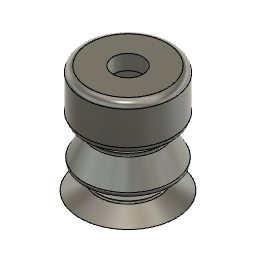
StyloVentouse v8 (Autodesk Fusion 360 archive; units mm, degrees)
design "VENTOUSE_15MM"
Autodesk Fusion 360 part; units mm, degrees
note: some values were not read from the file. Chosen so that the rebuilt part matches the saved one: which face or edge a step refers to; where a thread starts. Set by a fixed rule: which sketch regions a step uses.
sketch "Sketch1" plane through (0, 0, 0) normal (0, 1, 0) x (1, 0, 0)
sketch "Sketch2" plane through (0, 0, 0) normal (1, 0, 0) x (0, 0, -1)
  line L0 (8, 0) -> (4.6728, 1.6982)
  line L1 (4.6728, 1.6982) -> (7.5, 4.5279)
  line L2 (7.5, 4.5279) -> (5.2639, 9)
  line L3 (5.2639, 9) -> (7.5, 11)
  line L4 (7.5, 11) -> (7.5, 18)
  line L5 (7.5, 18) -> (2.5, 18)
  line L6 (2.5, 18) -> (2.5, 15.5)
  line L7 (2.5, 15.5) -> (4, 15.5)
  line L8 (4, 15.5) -> (4, 13.2)
  line L9 (4, 13.2) -> (2.5, 13.2)
  line L10 (2.5, 13.2) -> (2.5, 9)
  line L11 (2.5, 9) -> (6.2834, 4.725)
  line L12 (6.2834, 4.725) -> (4, 1.6283)
  line L13 (4, 1.6283) -> (8, 0)
  line L14 (0, 0) -> (0, 19.3777) construction
  dimension "d1" = 7.5
  dimension "d2" = 2.5
  dimension "d3" = 8
  dimension "d5" = 18
  dimension "d6" = 2.3
  dimension "d8" = 3
  dimension "d9" = 5
  dimension "d10" = 4
  dimension "d11" = 7
  dimension "d14" = 2.5
  dimension "d15" = 4
  dimension "d19" = 2
  dimension "d20" = 1
  dimension "d21" = 4
  dimension "d22" = 0.5
  dimension "d23" = 0.3681
  dimension "d24" = 1
  constraint vertical L4
  constraint perpendicular L4 L5
  constraint perpendicular L5 L6
  constraint perpendicular L6 L7
  constraint perpendicular L7 L8
  constraint perpendicular L8 L9
  constraint perpendicular L9 L10
  constraint collinear L6 L10
  constraint horizontal L0.start L14.start
  constraint horizontal L2.end L10.end
  constraint vertical L1.end L3.end
  constraint coincident L14.start origin
  constraint vertical L14
  measures "d1" distance of L14.start L4
  measures "d2" distance of L14.start L6
  measures "d3" distance of L0.start L14.start
  measures "d5" distance of L14.start L5
  measures "d6" distance of L7.end L8.end
  measures "d8" distance of L2.end L3.end
  measures "d9" distance of L1.end L2.end
  measures "d10" distance of L0.end L1.end
  measures "d11" distance of L3.end L4.end
  measures "d14" distance of L5.end L6.end
  measures "d15" distance of L8 L14.start
  measures "d19" vertical distance of L2.end L3.end
  measures "d20" distance of L2 L11.end
  measures "d21" horizontal distance of L12.end L14.start
  measures "d22" distance of L0.end L12
  measures "d23" distance of L0 L12.end
  measures "d24" distance of L1 L11.end
revolve "Revolve1" add sketch "Sketch2" angle 360 about axis through (0, 0, 0) along (0, 1, 0)
fillet "Fillet1" radius 1 1 edges at (-6.9925, 18, -2.7121)
fillet "Fillet2" radius 1 1 edges at (-6.9925, 11, -2.7121)
fillet "Fillet2" radius 0.5 1 edges at (-6.9925, 4.5279, -2.7121)
fillet "Fillet3" radius 0.25 1 edges at (-4.3565, 1.6982, -1.6897)
fillet "Fillet4" radius 0.5 1 edges at (-4.9077, 9, -1.9035)

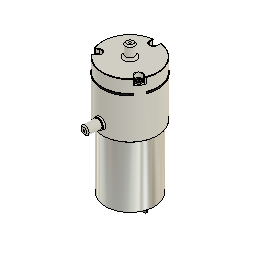
design "MICRO-POMPE 370"
Autodesk Fusion 360 part; units mm, degrees
sketch "Sketch1" plane through (0, 0, 0) normal (0, 0, 1) x (1, 0, 0)
  circle A0 centre (0, 0) radius 12.05
  dimension "d1" = 24.1
  measures "d1" diameter of A0
extrude "Extrude1" add sketch "Sketch1" along normal blind 30.9 makes body 1 in component "MOTEUR"
sketch "Sketch1 (2)" plane through (0, 0, 0) normal (0, 0, -1) x (1, 0, 0) in component "MOTEUR"
  circle A0 centre (0, 0) radius 12.05
  circle A1 centre (0, 0) radius 11.55
  dimension "d4" = 0.5
  measures "d4" distance of A0 A1
extrude "Extrude2" cut sketch "Sketch1 (2)" against normal blind 0.8 contours A1 bodies 1 in component "MOTEUR"
sketch "Sketch2" plane through (0, 0, 0.8) normal (0, 0, -1) x (1, 0, 0) in component "MOTEUR"
  circle A0 centre (0, 0) radius 11.55
  circle A1 centre (0, 0) radius 3.3
  dimension "d7" = 6.6
  measures "d7" diameter of A1
extrude "Extrude3" add sketch "Sketch2" along normal blind 2.3 contours A1 bodies 1 in component "MOTEUR"
fillet "Fillet1" radius 1 1 edges at (-3.0767, 1.1933, -1.5) on bodies 1 in component "MOTEUR"
sketch "Sketch3" plane through (0, 0, 0.8) normal (0, 0, -1) x (1, 0, 0) in component "MOTEUR"
  circle A0 centre (0, 0) radius 3.3
  circle A1 centre (0, 0) radius 11.55
  line L0 (0, 0) -> (9, 0) construction
  line L1 (10.8, -2) -> (10.8, 2)
  arc A2 (10.8, 2) -> (7.2, 2) centre (9, 2) ccw
  line L2 (7.2, 2) -> (7.2, -2)
  arc A3 (7.2, -2) -> (10.8, -2) centre (9, -2) ccw
  line L3 (9, -2) -> (9, 2) construction
  dimension "d11" = 9
  dimension "d12" = 4
  dimension "d13" = 1.8
  measures "d11" distance of A0.centre
  measures "d13" radius of A2
extrude "Extrude1'" add sketch "Sketch3" along normal blind 0.5 separate body contours L1 A2 L2 A3 makes body 2 in component "PAD_MOTEUR"
mirror "MirrorComponent1" about plane through (0, 0, 0) normal (0, 0, 1) of bodies 2 makes body 3 in component "PAD_MOTEUR(Mirror)"
sketch "Sketch4" plane through (0, 0, 0.8) normal (0, 0, -1) x (1, 0, 0) in component "MOTEUR"
  circle A0 centre (0, 0) radius 3.3
  circle A1 centre (0, 0) radius 11.55
  line L0 (-8, -2) -> (-10, -2)
  line L1 (-10, -2) -> (-10, -1.5)
  line L2 (-10, -1.5) -> (-8, -1.5)
  line L3 (-8, -1.5) -> (-8, -2)
  line L4 (-8, -2) -> (-10, -1.5) construction
  line L5 (-10, -2) -> (-8, -1.5) construction
  arc A2 (-7.2, 2) -> (-10.8, 2) centre (-9, 2) ccw
  line L6 (-9, -1.75) -> (-9, 3.8)
  dimension "d16" = 0.5
  dimension "d17" = 2
extrude "Extrude1''" add sketch "Sketch4" along normal blind 4 separate body contours L0 L1 L2 L3 makes body 4 in component "PIN"
fillet "Fillet1'" radius 0.5 2 edges at (-8, 1.75, -3.2) (-10, 1.75, -3.2) on bodies 4 in component "PIN"
other "C-Pattern1" in component "MOTEUR"
sketch "Sketch2 (2)" plane through (0, 0, 30.9) normal (0, 0, 1) x (-1, 0, 0)
  circle A0 centre (0, 0) radius 12.05
  circle A1 centre (0, 0) radius 13.55
  dimension "d23" = 27.1
  measures "d23" diameter of A1
extrude "Extrude1'''" add sketch "Sketch2 (2)" along normal blind 27.1 separate body contours A0 | A1 makes body 5 in component "CORPS"
sketch "Sketch1 (3)" plane through (0, 0, 58) normal (0, 0, 1) x (-1, 0, 0) in component "CORPS"
  circle A0 centre (0, 0) radius 13.55
  line L0 (0, 0) -> (0, -13.55) construction
  line L1 (1.75, -13.55) -> (1.75, -11.55)
  arc A1 (1.75, -11.55) -> (-1.75, -11.55) centre (0, -11.55) ccw
  line L2 (-1.75, -11.55) -> (-1.75, -13.55)
  arc A2 (-1.75, -13.55) -> (1.75, -13.55) centre (0, -13.55) ccw
  line L3 (0, -13.55) -> (0, -11.55) construction
  dimension "d26" = 2
  dimension "d27" = 3.5
  measures "d27" distance of L1 L2
extrude "Extrude2'" cut sketch "Sketch1 (3)" against normal blind 3 contours A0 L1 A1 L2 picked at (0.1949, -12.2125) bodies 5 in component "CORPS"
pattern_circular "C-Pattern1'" count 3 over 360 about axis through (0, 0, 30.9) along (0, 0, 1) of "Extrude2'" in component "CORPS"
sketch "Sketch2 (3)" plane through (0, 0, 58) normal (0, 0, 1) x (-1, 0, 0) in component "CORPS"
  line L0 (-10.7614, 8.2338) -> (-9.1276, 7.2905)
  arc A0 (-10.8776, 4.2595) -> (-9.1276, 7.2905) centre (-10.0026, 5.775) ccw
  line L1 (-10.8776, 4.2595) -> (-12.5114, 5.2027)
  arc A1 (-12.5114, 5.2027) -> (-1.75, -13.4365) centre (0, 0) ccw
  line L2 (-1.75, -13.4365) -> (-1.75, -11.55)
  arc A2 (1.75, -11.55) -> (-1.75, -11.55) centre (0, -11.55) ccw
  line L3 (1.75, -11.55) -> (1.75, -13.4365)
  arc A3 (1.75, -13.4365) -> (12.5114, 5.2027) centre (0, 0) ccw
  line L4 (12.5114, 5.2027) -> (10.8776, 4.2595)
  arc A4 (9.1276, 7.2905) -> (10.8776, 4.2595) centre (10.0026, 5.775) ccw
  line L5 (9.1276, 7.2905) -> (10.7614, 8.2338)
  arc A5 (10.7614, 8.2338) -> (-10.7614, 8.2338) centre (0, 0) ccw
  circle A6 centre (0, 0) radius 2.15
  dimension "d32" = 4.3
  measures "d32" diameter of A6
extrude "Extrude3'" add sketch "Sketch2 (3)" along normal blind 6.1 contours A6 bodies 5 in component "CORPS"
sketch "Sketch3 (2)" plane through (0, 0, 64.1) normal (0, 0, 1) x (-1, 0, 0) in component "CORPS"
  circle A0 centre (0, 0) radius 2.15
  circle A1 centre (0, 0) radius 0.5
  dimension "d35" = 1
  measures "d35" diameter of A1
extrude "Extrude4" cut sketch "Sketch3 (2)" against normal blind 6 contours A1 bodies 5 in component "CORPS"
fillet "Fillet1''" radius 1 1 edges at (2.0045, -0.7775, 58) on bodies 5 in component "CORPS"
fillet "Fillet2" radius 0.4 6 edges at (10.7614, -8.2338, 56.5) (12.5114, -5.2027, 56.5) (-10.7614, -8.2338, 56.5) (-12.5114, -5.2027, 56.5) (-1.75, 13.4365, 56.5) (1.75, 13.4365, 56.5) on bodies 5 in component "CORPS"
sketch "Sketch4 (2)" plane through (0, 0, 55) normal (0, 0, 1) x (-1, 0, 0) in component "CORPS"
  arc A0 (-2.2154, -13.3677) -> (2.2154, -13.3677) centre (0, 0) ccw
  arc A1 (1.75, -12.973) -> (2.2154, -13.3677) centre (2.15, -12.973) ccw
  line L0 (1.75, -12.973) -> (1.75, -11.55)
  arc A2 (1.75, -11.55) -> (-1.75, -11.55) centre (0, -11.55) ccw
  line L1 (-1.75, -11.55) -> (-1.75, -12.973)
  arc A3 (-2.2154, -13.3677) -> (-1.75, -12.973) centre (-2.15, -12.973) ccw
  circle A4 centre (0, -11.55) radius 1.5
  dimension "d41" = 3
  measures "d41" diameter of A4
extrude "Extrude1''''" add sketch "Sketch4 (2)" along normal blind 1.2 separate body contours A4 makes body 6 in component "VIS"
sketch "Sketch1 (4)" plane through (0, 0, 56.2) normal (0, 0, 1) x (-1, 0, 0) in component "VIS"
  circle A0 centre (0, -11.55) radius 1.5
  line L0 (-0.2169, -12.6709) -> (0.2169, -12.6709)
  line L1 (0.2169, -12.6709) -> (0.2169, -10.4291)
  line L2 (0.2169, -10.4291) -> (-0.2169, -10.4291)
  line L3 (-0.2169, -10.4291) -> (-0.2169, -12.6709)
  line L4 (-0.2169, -12.6709) -> (0.2169, -10.4291) construction
  line L5 (0.2169, -12.6709) -> (-0.2169, -10.4291) construction
  line L6 (-1.113, -11.7669) -> (1.113, -11.7669)
  line L7 (1.113, -11.7669) -> (1.113, -11.3331)
  line L8 (1.113, -11.3331) -> (-1.113, -11.3331)
  line L9 (-1.113, -11.3331) -> (-1.113, -11.7669)
  line L10 (-1.113, -11.7669) -> (1.113, -11.3331) construction
  line L11 (1.113, -11.7669) -> (-1.113, -11.3331) construction
extrude "Extrude2''" cut sketch "Sketch1 (4)" against normal blind 0.35 contours L0 L1 L3 L6 | L3 L6 L8 L9 | L1 L3 L6 L8 | L1 L6 L7 L8 | L1 L2 L3 L8 bodies 6 in component "VIS"
fillet "Fillet1'''" radius 0.2 2 edges at (1.3985, 12.0924, 55) (1.3985, 12.0924, 56.2) on bodies 6 in component "VIS"
other "C-Pattern1''" in component "CORPS"
ref_plane "WorkPlane1" through (0, 0, 12.125) normal (0.087156, 0.996195, 0) x (0, 0, 1) in component "CORPS"
sketch "Sketch5" plane through (0, 0, 12.125) normal (0.087156, 0.996195, 0) x (0, 0, 1) in component "CORPS"
  line L0 (18.775, -13.55) -> (18.775, 13.55)
  line L1 (18.775, 0) -> (23.775, 0) construction
  circle A0 centre (23.775, 0) radius 2.6631
  dimension "d50" = 5
  dimension "d51" = 5.3262
  measures "d50" distance of origin
  measures "d51" diameter of A0
extrude "Extrude5" add sketch "Sketch5" against normal blind 14.5 bodies 5 in component "CORPS"
sketch "Sketch6" plane through (-1.2638, -14.4448, 0) normal (-0.087156, -0.996195, 0) x (0.996195, -0.087156, 0) in component "CORPS"
  circle A0 centre (0, 35.9) radius 2.6631
  circle A1 centre (0, 35.9) radius 2.1
  circle A2 centre (0, 35.9) radius 0.5
  dimension "d54" = 4.2
  dimension "d55" = 1
  measures "d54" diameter of A1
  measures "d55" diameter of A2
extrude "Extrude6" add sketch "Sketch6" along normal blind 6.5 contours A1 bodies 5 in component "CORPS"
chamfer "Chamfer1" distance 0.6 angle 45 2 edges at (2.0045, 0.7775, 64.1) (-3.7807, -20.7494, 35.1406) on bodies 5 in component "CORPS"
fillet "Fillet3" radius 0.1 1 edges at (-0.3044, -14.5288, 33.4171) on bodies 5 in component "CORPS"
fillet "Fillet4" radius 0.2 19 edges at (10.5536, -8.277, 58) (9.7438, -7.6463, 58) (8.487, -4.9, 58) (11.4938, -4.6152, 58) (12.4449, -5.0011, 58) (11.7346, 6.775, 58) (1.8913, 13.2781, 58) (1.75, 12.2615, 58) (0, 9.8, 58) (-1.75, 12.2615, 58) (-1.8913, 13.2781, 58) (-11.7346, 6.775, 58) (-12.4449, -5.0011, 58) (-11.4938, -4.6152, 58) (-8.487, -4.9, 58) (-9.7438, -7.6463, 58) (-10.5536, -8.277, 58) (0, -13.55, 58) (12.633, 4.8999, 30.9) on bodies 5 in component "CORPS"
ref_plane "WorkPlane2" through (0, -0.0822, 50.8) normal (0, 0, 1) x (-1, 0, 0) in component "CORPS"
sketch "Sketch8" plane through (0, -0.0822, 50.8) normal (0, 0, 1) x (1, 0, 0) in component "CORPS"
  circle A0 centre (0, 0.0822) radius 13.65
  line L0 (0, 0.0822) -> (-12.7781, -4.7182)
  line L1 (0, 0.0822) -> (-2.2317, 13.5486)
  dimension "d61" = 27.3
  measures "d61" diameter of A0
extrude "Extrude1'''''" add sketch "Sketch8" along normal blind 1 separate body contours A0 L0 L1 picked at (-8.7073, -2.4762) makes body 7 in component "JOINT"
fillet "Fillet1''''" radius 0.1 2 edges at (-11.8212, 6.825, 51.8) (-11.8212, 6.825, 50.8) on bodies 7 in component "JOINT"
other "C-Pattern2" in component "CORPS"
component "MOTEUR" placed x (1, 0, 0) y (0, 1, 0) z (0, 0, 1) at (0, 0, 0)
component "CORPS" placed x (1, 0, 0) y (0, 1, 0) z (0, 0, 1) at (0, 0, 0)
component "PAD_MOTEUR" placed x (1, 0, 0) y (0, 1, 0) z (0, 0, 1) at (0, 0, 0) in component "MOTEUR"
component "PAD_MOTEUR(Mirror)" placed x (-1, 0, 0) y (0, 1, 0) z (0, 0, -1) at (0, 0, 0) in component "MOTEUR"
component "PIN" placed x (1, 0, 0) y (0, 1, 0) z (0, 0, 1) at (0, 0, 0) in component "MOTEUR"
component "PIN" placed x (-1, 0, 0) y (0, -1, 0) z (0, 0, 1) at (0, 0, 0) in component "MOTEUR"
component "VIS" placed x (1, 0, 0) y (0, 1, 0) z (0, 0, 1) at (0, 0, 0) in component "CORPS"
component "VIS" placed x (-0.5, 0.866025, 0) y (-0.866025, -0.5, 0) z (0, 0, 1) at (0, 0, 0) in component "CORPS"
component "VIS" placed x (-0.5, -0.866025, 0) y (0.866025, -0.5, 0) z (0, 0, 1) at (0, 0, 0) in component "CORPS"
component "JOINT" placed x (1, 0, 0) y (0, 1, 0) z (0, 0, 1) at (0, 0, 0) in component "CORPS"
component "JOINT" placed x (-0.5, 0.866025, 0) y (-0.866025, -0.5, 0) z (0, 0, 1) at (0, 0, 0) in component "CORPS"
component "JOINT" placed x (-0.5, -0.866025, 0) y (0.866025, -0.5, 0) z (0, 0, 1) at (0, 0, 0) in component "CORPS"
equation "d52 = -( ( 27 / 2 ) * 1 mm ) - 1 mm"

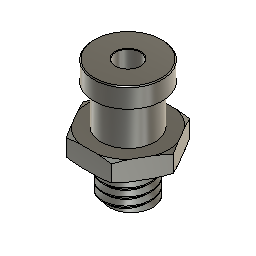
design "RACCORD-VENTOUSE"
Autodesk Fusion 360 part; units mm, degrees
sketch "Sketch1" plane through (0, 0, 0) normal (1, 0, 0) x (0, 1, 0)
  line L0 (0, 0) -> (3.5, 0)
  line L1 (3.5, 0) -> (3.5, -2)
  line L2 (3.5, -2) -> (2.75, -2)
  line L3 (2.75, -2) -> (2.75, -6)
  line L4 (2.75, -6) -> (0, -6)
  line L5 (0, -6) -> (0, 0)
  dimension "d1" = 3.5
  dimension "d2" = 2.75
  dimension "d3" = 2
  dimension "d4" = 4
  measures "d1" distance of L0.start
  measures "d2" distance of L3 L5
revolve "Revolve1" add sketch "Sketch1" angle 360 about axis through (0, 0, -6) along (0, 0, 1)
sketch "Sketch2" plane through (0, 0, -6) normal (0, 0, -1) x (1, 0, 0)
  circle A0 centre (0, 0) radius 2.75
  line L0 (2.3094, -4) -> (4.6188, 0)
  line L1 (4.6188, 0) -> (2.3094, 4)
  line L2 (2.3094, 4) -> (-2.3094, 4)
  line L3 (-2.3094, 4) -> (-4.6188, 0)
  line L4 (-4.6188, 0) -> (-2.3094, -4)
  line L5 (-2.3094, -4) -> (2.3094, -4)
  dimension "d6" = 8
  measures "d6" distance of L2 L5
extrude "Extrude1" add sketch "Sketch2" along normal blind 2 contours A0 | L0 L1 L2 L3 L4 L5
sketch "Sketch3" plane through (0, 0, 0) normal (0, 1, 0) x (1, 0, 0)
  line L0 (4.6188, 6) -> (2.3094, 6) construction
  line L1 (4.6188, 6) -> (4.6188, 8) construction
  line L2 (4.1193, 6) -> (4.6188, 6.1563)
  line L3 (4.6188, 6) -> (4.1193, 6)
  line L4 (4.6188, 8) -> (2.3094, 8) construction
  line L5 (4.6188, 7.8437) -> (4.1193, 8)
  line L6 (4.1193, 8) -> (4.6188, 8)
  line L7 (4.6188, 7.8437) -> (4.6188, 8)
  line L8 (4.6188, 6) -> (4.6188, 6.1563)
revolve "Revolve2" cut sketch "Sketch3" angle 360 about axis through (0, 0, 1.75) along (0, 0, 1)
chamfer "Chamfer1" distance 0.1 angle 45 1 edges at (-3.2631, 1.2657, 0)
sketch "Sketch4" plane through (0, 0, -8) normal (0, 0, -1) x (1, 0, 0)
  arc A0 (-3.9563, 1.1475) -> (-3.9563, -1.1475) centre (0, 0) ccw
  line L0 (-3.9563, -1.1475) -> (-2.9719, -2.8525)
  arc A1 (-2.9719, -2.8525) -> (-0.9843, -4) centre (0, 0) ccw
  line L1 (-0.9843, -4) -> (0.9843, -4)
  arc A2 (0.9843, -4) -> (2.9719, -2.8525) centre (0, 0) ccw
  line L2 (2.9719, -2.8525) -> (3.9563, -1.1475)
  arc A3 (3.9563, -1.1475) -> (3.9563, 1.1475) centre (0, 0) ccw
  line L3 (3.9563, 1.1475) -> (2.9719, 2.8525)
  arc A4 (2.9719, 2.8525) -> (0.9843, 4) centre (0, 0) ccw
  line L4 (0.9843, 4) -> (-0.9843, 4)
  arc A5 (-0.9843, 4) -> (-2.9719, 2.8525) centre (0, 0) ccw
  line L5 (-2.9719, 2.8525) -> (-3.9563, 1.1475)
  circle A6 centre (0, 0) radius 2
  dimension "d11" = 4
  measures "d11" diameter of A6
extrude "Extrude2" add sketch "Sketch4" along normal blind 4 contours A6
sketch "Sketch5" plane through (0, 0, -12) normal (0, 0, -1) x (1, 0, 0)
  circle A0 centre (0, 0) radius 2
  circle A1 centre (0, 0) radius 1.25
  dimension "d14" = 2.5
  measures "d14" diameter of A1
extrude "Extrude3" cut sketch "Sketch5" against normal through all contours A1
chamfer "Chamfer2" distance 0.05 angle 45 1 edges at (-1.1654, 0.452, 0)
chamfer "Chamfer3" distance 0.5 angle 45 1 edges at (-1.1654, -0.452, -12)
sketch "Sketch6" plane through (0, 0, -12) normal (0, 0, -1) x (1, 0, 0)
  circle A0 centre (0, 0) radius 2
  circle A1 centre (0, 0) radius 1.75
  circle A2 centre (0, 0) radius 2.05
  dimension "d18" = 4.1
  measures "d18" diameter of A2
extrude "Extrude4" add sketch "Sketch6" against normal blind 3 contours A2
thread "Thread1" "ISO Metric profile 5.0 M5x0.8 6g" major diameter 4.901 minor diameter 3.9895 pitch 0.8 angle 60 modelled right hand crest width 0.1 on face at (2.0475, 0.1022, -10) crest through (2.4505, 0, -12.05)
equation "d1 = ( 7 / 2 ) * 1 mm"
equation "d2 = ( 5.5 / 2 ) * 1 mm"
